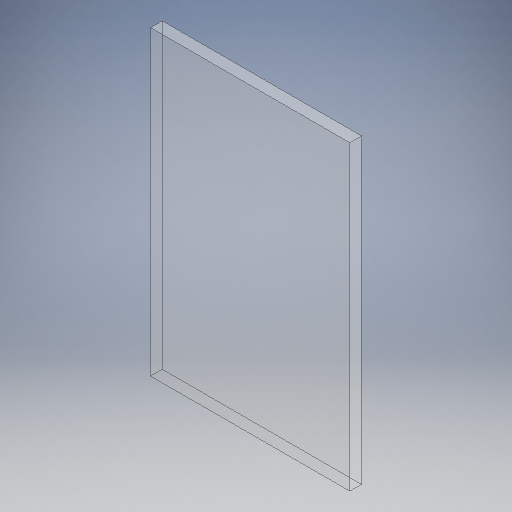
# Autodesk Inventor part: cowl_front
Saved by Autodesk Inventor 2025.2 (Build 292293000, 293)
## iProperties
Created: 2025-02-07
Part Number: cowl_front
Material: 폴리카보네이트, 선명
Document SubType Name: Modeling
Designer: jbhma
Density: 1.2 g/cm^3
Appearance: 폴리카보네이트 - 선명
Author: jbhma
Autodesk Inventor part; units mm, degrees
ref_plane "YZ Plane" through (0, 0, 0) normal (1, 0, 0) x (0, 1, 0)
ref_plane "XZ Plane" through (0, 0, 0) normal (0, 1, 0) x (-1, 0, 0)
ref_plane "XY Plane" through (0, 0, 0) normal (0, 0, 1) x (1, 0, 0)
sketch "스케치1" plane through (0, 0, 0) normal (0, 0, 1) x (1, 0, 0)
  line L0 (0, 0) -> (340, 0)
  line L1 (340, 0) -> (340, -515)
  line L2 (340, -515) -> (0, -515)
  line L3 (0, -515) -> (0, 0)
  dimension "d0" = 340
  dimension "d1" = 515
  constraints: 8 end point, 2 parallel, 1 horizontal, 1 perpendicular
  measures "d0" distance of L1.end L2.end
  measures "d1" distance of L0.end L1.end
extrude "돌출1" add sketch "스케치1" along normal blind 20
